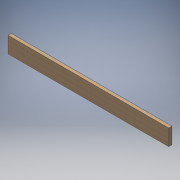
# Autodesk Inventor part: Балка
Saved by Autodesk Inventor 2019 (Build 230136000, 136)
## iProperties
Created: 2018-10-11
Part Number: Балка
Material: Ясень
Document SubType Name: Modeling
Designer: Андреев Н.Л.
Density: 0.641 g/cm^3
Appearance: Дверь — ясень
Mass: 10204.7 g
Surface Area: 9712 cm^2
Volume: 15920 cm^3
ДЛИНА: 1990
ШИРИНА: 200
ТОЛЩВЫС: 40
Author: Андреев Н.Л.
Autodesk Inventor part; units mm, degrees
ref_plane "YZ Plane" through (0, 0, 0) normal (1, 0, 0) x (0, 1, 0)
ref_plane "XZ Plane" through (0, 0, 0) normal (0, 1, 0) x (-1, 0, 0)
ref_plane "XY Plane" through (0, 0, 0) normal (0, 0, 1) x (1, 0, 0)
sketch "Эскиз1" plane through (0, 0, 0) normal (0, 0, 1) x (1, 0, 0)
  line L0 (1990, 325) -> (1990, 125) construction
  line L1 (1990, 325) -> (1950, 325) construction
  line L2 (1950, 125) -> (1950, 325) construction
  line L3 (1990, 125) -> (1950, 125) construction
  line L4 (1990, 325) -> (0, 325)
  line L5 (0, 325) -> (0, 125)
  line L6 (0, 125) -> (1990, 125)
  line L7 (1990, 125) -> (1990, 325)
  line L8 (0, 125) -> (0, 325) construction
  line L9 (0, 125) -> (40, 125) construction
  line L10 (40, 325) -> (40, 125) construction
  line L11 (0, 325) -> (40, 325) construction
  constraints: 8 end point, 2 parallel, 1 horizontal, 1 perpendicular
extrude "Выдавливание1" add sketch "Эскиз1" against normal blind 40
